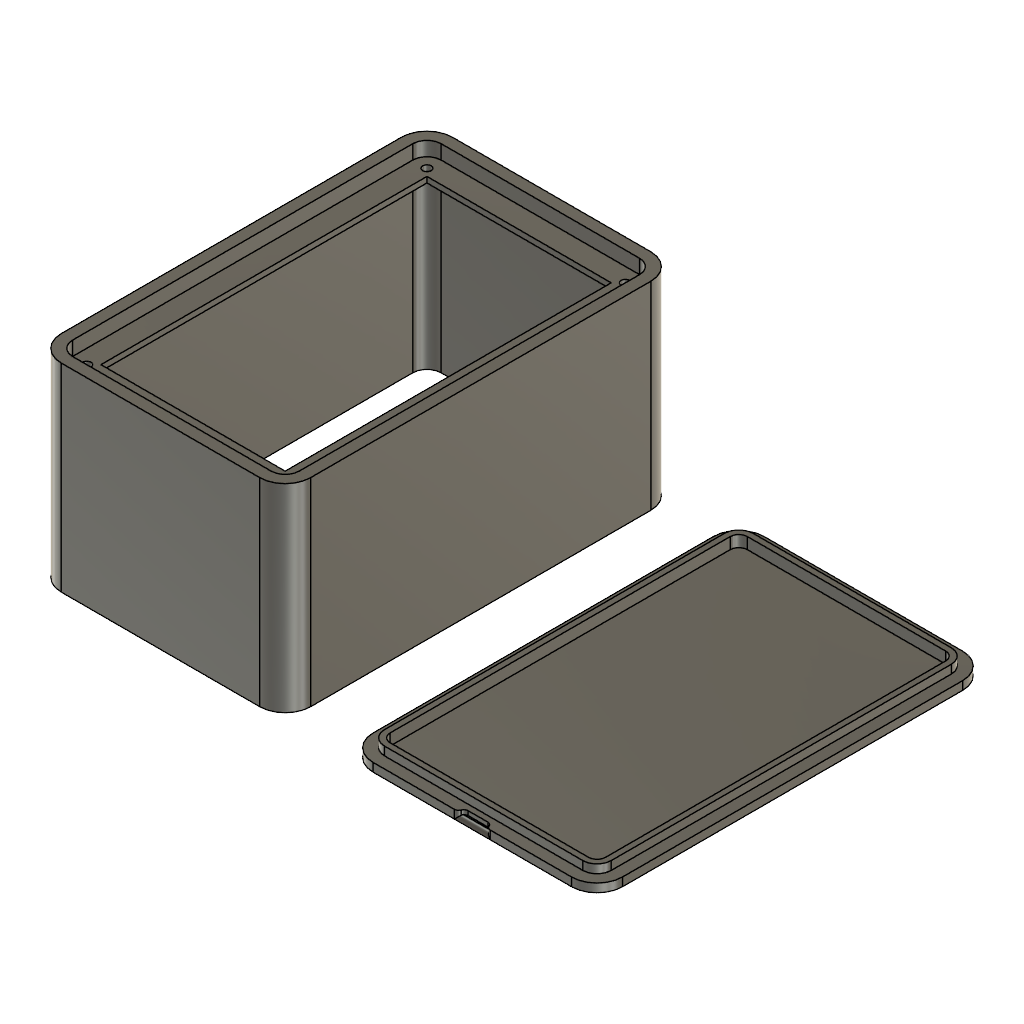
biometric scanner enclosure (Autodesk Fusion 360 design; units mm, degrees)
part number: 2026-09-12-10-18-39-435
Autodesk Fusion 360 part; units mm, degrees
note: some values were not read from the file. Chosen so that the rebuilt part matches the saved one: which face or edge a step refers to; which pieces of a blend or face edit are solid.
sketch "Sketch1" plane through (0, 0, 0) normal (0, 0, 1) x (1, 0, 0)
  line L0 (-35, 65) -> (35, 65)
  line L1 (40, 60) -> (40, -60)
  line L2 (35, -65) -> (-35, -65)
  line L3 (-40, -60) -> (-40, 60)
  arc A0 (-35, 65) -> (-40, 60) centre (-35, 60) ccw
  arc A1 (40, 60) -> (35, 65) centre (35, 60) ccw
  arc A2 (-40, -60) -> (-35, -65) centre (-35, -60) ccw
  arc A3 (35, -65) -> (40, -60) centre (35, -60) ccw
  point P0 (-40, 65)
  point P1 (40, 65)
  point P2 (-40, -65)
  dimension "d1" = 80
  dimension "d2" = 130
  dimension "d3" = 40
  dimension "d4" = 65
  dimension "d5" = 5
  dimension "d6" = 5
  dimension "d7" = 5
  dimension "d8" = 5
  constraint horizontal L0
  constraint vertical L1
  constraint horizontal L2
  constraint vertical L3
  constraint coincident P0 L0
  constraint coincident P0 L3
  constraint tangent L0 A0
  constraint tangent L3 A0
  constraint coincident P1 L0
  constraint coincident P1 L1
  constraint tangent L0 A1
  constraint tangent L1 A1
  constraint coincident P2 L2
  constraint coincident P2 L3
  constraint tangent L2 A2
  constraint tangent L3 A2
  constraint tangent L1 A3
  constraint tangent L2 A3
  measures "d1" distance of P0 P1
  measures "d2" distance of P0 P2
  measures "d3" distance of origin L3
  measures "d4" distance of origin L0
  measures "d5" radius of A0
  measures "d6" radius of A1
  measures "d7" radius of A2
  measures "d8" radius of A3
extrude "Extrude1" add sketch "Sketch1" along normal blind 70 makes body 1
shell "Shell1" thickness 4 outward yes removed faces 2 at (-13.3333, 20, 0) at (-13.3333, 20, 70) on bodies 1
sketch "Sketch2" plane through (0, 0, 70) normal (0, 0, 1) x (-1, 0, 0)
  line L0 (40, 60) -> (40, -60)
  arc A0 (35, -65) -> (40, -60) centre (35, -60) ccw
  line L1 (35, -65) -> (-35, -65)
  arc A1 (-40, -60) -> (-35, -65) centre (-35, -60) ccw
  line L2 (-40, -60) -> (-40, 60)
  arc A2 (-35, 65) -> (-40, 60) centre (-35, 60) ccw
  line L3 (-35, 65) -> (35, 65)
  arc A3 (40, 60) -> (35, 65) centre (35, 60) ccw
  arc A4 (44, 60) -> (35, 69) centre (35, 60) ccw
  line L4 (35, 69) -> (-35, 69)
  arc A5 (-35, 69) -> (-44, 60) centre (-35, 60) ccw
  line L5 (-44, 60) -> (-44, -60)
  arc A6 (-44, -60) -> (-35, -69) centre (-35, -60) ccw
  line L6 (-35, -69) -> (35, -69)
  arc A7 (35, -69) -> (44, -60) centre (35, -60) ccw
  line L7 (44, -60) -> (44, 60)
  line L8 (-40, -65) -> (40, -65)
  line L9 (40, -65) -> (40, 65)
  line L10 (40, 65) -> (-40, 65)
  line L11 (-40, 65) -> (-40, -65)
  line L12 (35, 60) -> (-35, 60)
  line L13 (-35, 60) -> (-35, -60)
  line L14 (-35, -60) -> (35, -60)
  line L15 (35, -60) -> (35, 60)
  line L16 (35, 60) -> (-35, -60) construction
  line L17 (-35, 60) -> (35, -60) construction
  line L18 (32.5, -57.5) -> (-32.5, -57.5)
  line L19 (-32.5, -57.5) -> (-32.5, 57.5)
  line L20 (-32.5, 57.5) -> (32.5, 57.5)
  line L21 (32.5, 57.5) -> (32.5, -57.5)
  circle A8 centre (35, 60) radius 1.5
  circle A9 centre (35, -60) radius 1.5
  circle A10 centre (-35, 60) radius 1.5
  circle A11 centre (-35, -60) radius 1.5
  dimension "d12" = 70
  dimension "d13" = 120
  dimension "d14" = 3
  dimension "d15" = 3
  dimension "d16" = 3
  dimension "d17" = 3
  dimension "d18" = 65
  dimension "d19" = 115
  dimension "d20" = 57.5
  dimension "d21" = 32.5
  constraint horizontal L8
  constraint vertical L9
  constraint horizontal L10
  constraint vertical L11
  constraint horizontal L12
  constraint perpendicular L12 L13
  constraint parallel L12 L14
  constraint parallel L13 L15
  constraint coincident L16 origin
  constraint coincident L17 origin
  constraint horizontal L18
  constraint vertical L19
  constraint horizontal L20
  constraint vertical L21
  constraint coincident A3.centre A4.centre
  constraint coincident A0.centre A7.centre
  constraint coincident A2.centre A5.centre
  constraint coincident A1.centre A6.centre
  measures "d12" distance of A1.centre A0.centre
  measures "d13" distance of A2.centre A1.centre
  measures "d14" diameter of A8
  measures "d15" diameter of A9
  measures "d16" diameter of A10
  measures "d17" diameter of A11
  measures "d18" distance of L18.start L18.end
  measures "d19" distance of L18.start L20.end
  measures "d20" distance of origin L18
  measures "d21" distance of origin L21
extrude "Extrude2" add sketch "Sketch2" against normal blind 2 separate body contours L0 A0 L1 A1 L2 A2 L3 A3 L8 L9 L10 L11 | L12 L13 L14 L15 A8 A9 A10 A11 makes body 2
move_body "Move1" bodies 2 to x (1, 0, 0) y (0, 1, 0) z (0, 0, 1) at (0, 0, -5)
extrude "Extrude3" add 1 faces at (-41.3333, 20, 0) along direction (0, 0, -1) blind 3 separate body on bodies 1 makes body 3
move_body "Move2" bodies 3 to x (1, 0, 0) y (0, 1, 0) z (0, 0, 1) at (110, 0, 3)
sketch "Sketch3" plane through (0, 0, 3) normal (0, 0, 1) x (-1, 0, 0)
  line L0 (-70, 60) -> (-70, -60)
  arc A0 (-75, -65) -> (-70, -60) centre (-75, -60) ccw
  line L1 (-75, -65) -> (-145, -65)
  arc A1 (-150, -60) -> (-145, -65) centre (-145, -60) ccw
  line L2 (-150, -60) -> (-150, 60)
  arc A2 (-145, 65) -> (-150, 60) centre (-145, 60) ccw
  line L3 (-145, 65) -> (-75, 65)
  arc A3 (-70, 60) -> (-75, 65) centre (-75, 60) ccw
  arc A4 (-66, 60) -> (-75, 69) centre (-75, 60) ccw
  line L4 (-75, 69) -> (-145, 69)
  arc A5 (-145, 69) -> (-154, 60) centre (-145, 60) ccw
  line L5 (-154, 60) -> (-154, -60)
  arc A6 (-154, -60) -> (-145, -69) centre (-145, -60) ccw
  line L6 (-145, -69) -> (-75, -69)
  arc A7 (-75, -69) -> (-66, -60) centre (-75, -60) ccw
  line L7 (-66, -60) -> (-66, 60)
  line L8 (-75, -65) -> (-145, -65)
  line L9 (-150, -60) -> (-150, 60)
  line L10 (-145, 65) -> (-75, 65)
  line L11 (-70, 60) -> (-70, -60)
  arc A8 (-75, -65) -> (-70, -60) centre (-75, -60) ccw
  arc A9 (-150, -60) -> (-145, -65) centre (-145, -60) ccw
  arc A10 (-70, 60) -> (-75, 65) centre (-75, 60) ccw
  arc A11 (-145, 65) -> (-150, 60) centre (-145, 60) ccw
  dimension "d26" = 5
  dimension "d27" = 5
  dimension "d28" = 5
  dimension "d29" = 5
  constraint horizontal L8
  constraint vertical L9
  constraint horizontal L10
  constraint vertical L11
  constraint tangent L8 A8
  constraint tangent L11 A8
  constraint tangent L8 A9
  constraint tangent L9 A9
  constraint tangent L10 A10
  constraint tangent L11 A10
  constraint tangent L9 A11
  constraint tangent L10 A11
  measures "d26" radius of A8
  measures "d27" radius of A9
  measures "d28" radius of A10
  measures "d29" radius of A11
extrude "Extrude4" add sketch "Sketch3" along normal blind 3 separate body contours L0 A0 L1 A1 L2 A2 L3 A3 L8 L9 L10 L11 A8 A9 A10 A11 makes body 4
extrude "Extrude5" add 1 faces at (96.6667, 20, 3) along direction (0, 0, -1) blind 3 on bodies 4 bodies 3 4
shell "Shell2" thickness 2 removed faces 1 at (96.6667, 20, 6) on bodies 3
sketch "Sketch4" plane through (0, 0, 0) normal (0, 0, -1) x (1, 0, 0)
  line L0 (-40, -60) -> (-40, 60)
  arc A0 (-35, 65) -> (-40, 60) centre (-35, 60) ccw
  line L1 (-35, 65) -> (35, 65)
  arc A1 (40, 60) -> (35, 65) centre (35, 60) ccw
  line L2 (40, 60) -> (40, -60)
  arc A2 (35, -65) -> (40, -60) centre (35, -60) ccw
  line L3 (35, -65) -> (-35, -65)
  arc A3 (-40, -60) -> (-35, -65) centre (-35, -60) ccw
  arc A4 (-35, 69) -> (-44, 60) centre (-35, 60) ccw
  line L4 (-44, 60) -> (-44, -60)
  arc A5 (-44, -60) -> (-35, -69) centre (-35, -60) ccw
  line L5 (-35, -69) -> (35, -69)
  arc A6 (35, -69) -> (44, -60) centre (35, -60) ccw
  line L6 (44, -60) -> (44, 60)
  arc A7 (44, 60) -> (35, 69) centre (35, 60) ccw
  line L7 (35, 69) -> (-35, 69)
  line L8 (-5, 67) -> (5, 67)
  line L9 (5, 67) -> (5, 63)
  line L10 (5, 63) -> (-5, 63)
  line L11 (-5, 63) -> (-5, 67)
  dimension "d35" = 45
  constraint horizontal L8
  constraint vertical L9
  constraint horizontal L10
  constraint vertical L11
  measures "d35" distance of L2 L11
extrude "Extrude6" cut sketch "Sketch4" against normal blind 5 contours L1 L8 L9 L11 | L1 L9 L10 L11 bodies 1
fillet "Fillet1" radius 2 4 edges at (-5, -67, 2.5) (-5, -65, 2.5) (5, -67, 2.5) (5, -65, 2.5) on bodies 1
sketch "Sketch5" plane through (0, 0, 3) normal (0, 0, 1) x (-1, 0, 0)
  line L0 (-70, 60) -> (-70, -60)
  arc A0 (-75, -65) -> (-70, -60) centre (-75, -60) ccw
  line L1 (-75, -65) -> (-145, -65)
  arc A1 (-150, -60) -> (-145, -65) centre (-145, -60) ccw
  line L2 (-150, -60) -> (-150, 60)
  arc A2 (-145, 65) -> (-150, 60) centre (-145, 60) ccw
  line L3 (-145, 65) -> (-75, 65)
  arc A3 (-70, 60) -> (-75, 65) centre (-75, 60) ccw
  arc A4 (-66, 60) -> (-75, 69) centre (-75, 60) ccw
  line L4 (-75, 69) -> (-145, 69)
  arc A5 (-145, 69) -> (-154, 60) centre (-145, 60) ccw
  line L5 (-154, 60) -> (-154, -60)
  arc A6 (-154, -60) -> (-145, -69) centre (-145, -60) ccw
  line L6 (-145, -69) -> (-75, -69)
  arc A7 (-75, -69) -> (-66, -60) centre (-75, -60) ccw
  line L7 (-66, -60) -> (-66, 60)
  line L8 (-105, 67) -> (-115, 67)
  line L9 (-115, 67) -> (-115, 71)
  line L10 (-115, 71) -> (-105, 71)
  line L11 (-105, 71) -> (-105, 67)
  dimension "d40" = 10
  dimension "d41" = 4
  dimension "d42" = 35
  constraint horizontal L8
  constraint vertical L9
  constraint horizontal L10
  constraint vertical L11
  measures "d40" distance of L8.start L8.end
  measures "d41" distance of L8.start L10.end
  measures "d42" distance of L2 L9
extrude "Extrude7" cut sketch "Sketch5" against normal blind 1.5 contours L4 L8 L9 L11 | L4 L9 L10 L11 bodies 3
fillet "Fillet2" radius 1.5 7 edges at (105, -69, 2.25) (110, -69, 1.5) (115, -69, 2.25) (115, -67, 2.25) (115, -68, 1.5) (105, -67, 2.25) (105, -68, 1.5) on bodies 3
